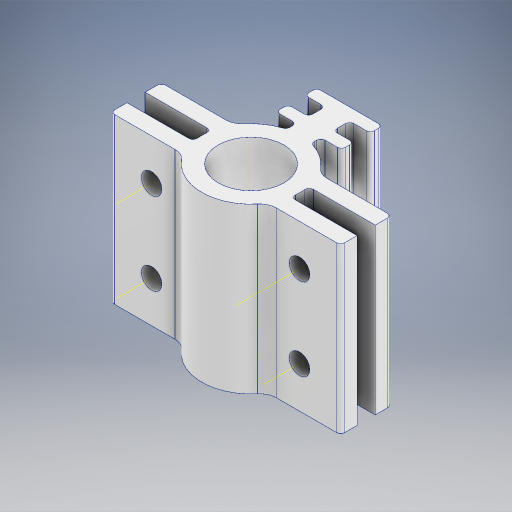
# Autodesk Inventor part: link7
Saved by Autodesk Inventor 2024.1 (Build 281209000, 209)
## iProperties
Created: 2023-09-09
Part Number: link7
Material: Aluminum 6061
Document SubType Name: Modeling
Designer: Camilo
Density: 2.7 g/cm^3
Appearance: Aluminum - Flat
Mass: 0.783285 g
Surface Area: 5.56806 cm^2
Volume: 0.290105 cm^3
Author: Camilo
Autodesk Inventor part; units mm, degrees
ref_plane "YZ Plane" through (0, 0, 0) normal (1, 0, 0) x (0, 1, 0)
ref_plane "XZ Plane" through (0, 0, 0) normal (0, 1, 0) x (-1, 0, 0)
ref_plane "XY Plane" through (0, 0, 0) normal (0, 0, 1) x (1, 0, 0)
sketch "Sketch2" plane through (0, 0, 0) normal (0, 1, 0) x (-1, 0, 0)
  circle A0 centre (0, 0) radius 4
  line L0 (-14, -10) -> (14, -10)
  line L1 (14, -10) -> (14, 10)
  line L2 (14, 10) -> (-14, 10)
  line L3 (-14, 10) -> (-14, -10)
  line L4 (-14, 0) -> (-14, -1.1)
  line L5 (-14, 0) -> (-14, 1.1)
  line L6 (14, 0) -> (14, -1.1)
  circle A1 centre (0, 0) radius 6
  line L7 (-14, -1.1) -> (-5.8983, -1.1)
  line L8 (-14, 1.1) -> (-5.8983, 1.1)
  line L9 (14, 0) -> (14, 1.1)
  line L10 (14, 1.1) -> (5.8983, 1.1)
  line L11 (14, -1.1) -> (5.8983, -1.1)
  line L12 (-14, -1.1) -> (-6.5, -1.1)
  line L13 (-14, -1.1) -> (-14, -3.1)
  line L14 (-14, -3.1) -> (-5.1371, -3.1)
  line L15 (-14, 1.1) -> (-14, 3.1)
  line L16 (-14, 3.1) -> (-5.1371, 3.1)
  line L17 (14, -1.1) -> (14, -3.1)
  line L18 (14, -3.1) -> (5.1371, -3.1)
  line L19 (14, 1.1) -> (14, 3.1)
  line L20 (14, 3.1) -> (5.1371, 3.1)
  point P0 (0, -10)
  dimension "d50" = 12
  dimension "d37" = 8
  dimension "d38" = 28
  dimension "d39" = 20
  dimension "d40" = 14
  dimension "d41" = 10
  dimension "d42" = 1.1
  dimension "d46" = 1.1
  dimension "d48" = 1.1
  dimension "d51" = 1.1
  dimension "d52" = 7.5
  dimension "d53" = 2
  dimension "d54" = 2
  dimension "d55" = 2
  dimension "d56" = 2
  constraints: 42 end point, 10 point on line, 5 perpendicular, 3 horizontal, 3 midpoint, 3 parallel, 2 coincident, 1 centre point, 10 other
  measures "d37" diameter of A0
  measures "d38" distance of L2.end L1.end
  measures "d39" distance of L1.end L0.end
  measures "d40" horizontal distance of point (0, 0) L0.start
  measures "d41" distance of point (0, -10) point (0, 0)
  measures "d42" distance of L4.start L4.end
  measures "d46" distance of L4.start L5.end
  measures "d48" distance of L6.start L6.end
  measures "d51" distance of L6.start L9.end
  measures "d52" distance of L4.end L12.end
  measures "d53" distance of L4.end L13.end
  measures "d54" distance of L5.end L15.end
  measures "d55" distance of L6.end L17.end
  measures "d56" distance of L9.end L19.end
extrude "Extrusion5" add sketch "Sketch2" along normal mid plane 20 contours L3 L7 A1 L14 | L18 A1 L11 L1 | A1 | L3 L16 A1 L8 | L10 A1 L20 L1
sketch "Sketch3" plane through (0, 0, 0) normal (0, 0, 1) x (1, 0, 0)
  line L0 (14, 10) -> (5.1371, 10) projected
  line L1 (14, 10) -> (9, 10)
  line L2 (9, 10) -> (9, 5)
  line L3 (9, 5) -> (14, 5)
  line L4 (14, 5) -> (14, 10)
  circle A0 centre (9, 5) radius 1.25
  line L5 (5.1371, 10) -> (-5.1371, 10) projected
  line L6 (0, 10) -> (0, -10)
  line L7 (4, -10) -> (-4, -10) projected
  line L8 (-14, -10) -> (-14, 10) projected
  line L9 (-14, 0) -> (14, 0)
  line L10 (14, -10) -> (14, 10) projected
  circle A1 centre (9, -5) radius 1.25
  circle A2 centre (-9, 5) radius 1.25
  circle A3 centre (-9, -5) radius 1.25
  point P0 (0, 0)
  dimension "d59" = 5
  dimension "d60" = 5
  dimension "d61" = 2.5
  constraints: 12 end point, 4 centre point, 4 midpoint, 3 symmetric about line, 2 parallel, 1 coincident, 1 horizontal, 1 perpendicular, 3 other
  measures "d59" distance of L3.end L2.end
  measures "d60" distance of L2.end L1.end
  measures "d61" diameter of A0
extrude "Extrusion6" cut sketch "Sketch3" along normal mid plane 20 contours A0 L3 L2 | L2 L3 A0 | A1 | A2 | A3
fillet "Face Fillet1" radius 2 1 edges at (5.1371, 0, -3.1)
fillet "Face Fillet2" radius 2 1 edges at (-5.1371, 0, -3.1)
fillet "Face Fillet3" radius 2 1 edges at (-5.1371, 0, 3.1)
fillet "Face Fillet4" radius 2 1 edges at (5.1371, 0, 3.1)
fillet "Face Fillet5" radius 0.5 1 edges at (-5.8983, 0, -1.1)
fillet "Face Fillet6" radius 0.5 1 edges at (-5.8983, 0, 1.1)
fillet "Face Fillet7" radius 0.5 1 edges at (5.8983, 0, -1.1)
fillet "Face Fillet8" radius 0.5 1 edges at (5.8983, 0, 1.1)
sketch "Sketch4" plane through (0, 10, 0) normal (0, 1, 0) x (1, 0, 0)
  circle A0 centre (0, 0) radius 6
  line L0 (0, 6) -> (0, 7)
  line L1 (0, 7) -> (1.5, 7)
  line L2 (0, 7) -> (-1.5, 7)
  line L3 (1.5, 7) -> (1.5, 5.8095)
  line L4 (-1.5, 7) -> (-1.5, 5.8095)
  line L5 (0, 7) -> (4, 7)
  line L6 (4, 7) -> (-4, 7)
  line L7 (-4, 7) -> (-4, 8.5)
  line L8 (-4, 8.5) -> (4, 8.5)
  line L9 (4, 8.5) -> (4, 7)
  line L10 (0, 8.5) -> (1.5, 8.5)
  line L11 (1.5, 8.5) -> (-1.5, 8.5)
  line L12 (-1.5, 8.5) -> (-1.5, 10.5)
  line L13 (-1.5, 10.5) -> (1.5, 10.5)
  line L14 (1.5, 10.5) -> (1.5, 8.5)
  line L15 (-1.5, 10.5) -> (-4, 10.5)
  line L16 (-4, 10.5) -> (4, 10.5)
  line L17 (4, 10.5) -> (4, 12)
  line L18 (4, 12) -> (-4, 12)
  line L19 (-4, 12) -> (-4, 10.5)
  dimension "d72" = 1
  dimension "d73" = 1.5
  dimension "d74" = 1.5
  dimension "d75" = 4
  dimension "d76" = 8
  dimension "d77" = 1.5
  dimension "d78" = 2
  dimension "d79" = 8
  dimension "d80" = 1.5
  dimension "d82" = 12
  constraints: 40 end point, 7 horizontal, 7 parallel, 3 perpendicular, 3 point on circle, 2 vertical, 1 centre point, 1 coincident, 1 midpoint, 1 point on line
  measures "d72" distance of L0.start L0.end
  measures "d73" distance of L0.end L1.end
  measures "d74" distance of L0.end L2.end
  measures "d75" distance of L0.end L5.end
  measures "d76" distance of L7.end L8.end
  measures "d77" distance of L6.end L7.end
  measures "d78" distance of L11.end L12.end
  measures "d79" distance of L18.end L17.end
  measures "d80" distance of L17.end L16.end
  measures "d82" diameter of A0
extrude "Extrusion7" add sketch "Sketch4" against normal blind 20 contours A0 L0 L1 L3 | L4 L2 L0 A0 | L1 L2 L6 L7 L8 L9 L5 | L8 L12 L13 L14 | L13 L15 L19 L18 L17 L16
fillet "Face Fillet9" radius 0.5 1 edges at (1.5, 0, -5.8095)
fillet "Face Fillet10" radius 0.5 1 edges at (1.5, 0, -7)
fillet "Face Fillet11" radius 0.5 1 edges at (-1.5, 0, -5.8095)
fillet "Face Fillet12" radius 0.5 1 edges at (-1.5, 0, -7)
fillet "Face Fillet13" radius 0.5 1 edges at (-1.5, 0, -8.5)
fillet "Face Fillet14" radius 0.5 1 edges at (-1.5, 0, -10.5)
fillet "Face Fillet15" radius 0.5 1 edges at (1.5, 0, -8.5)
fillet "Face Fillet16" radius 0.5 1 edges at (1.5, 0, -10.5)
fillet "Face Fillet17" radius 0.5 1 edges at (4, 0, -7)
fillet "Face Fillet18" radius 0.5 1 edges at (4, 0, -8.5)
fillet "Face Fillet19" radius 0.5 1 edges at (-4, 0, -8.5)
fillet "Face Fillet20" radius 0.5 1 edges at (-4, 0, -7)
fillet "Face Fillet21" radius 0.5 1 edges at (-4, 0, -10.5)
fillet "Face Fillet22" radius 0.5 1 edges at (-4, 0, -12)
fillet "Face Fillet23" radius 0.5 1 edges at (4, 0, -10.5)
fillet "Face Fillet24" radius 0.5 1 edges at (4, 0, -12)
fillet "Face Fillet25" radius 0.5 1 edges at (14, 0, 3.1)
fillet "Face Fillet26" radius 0.5 1 edges at (14, 0, -3.1)
fillet "Face Fillet27" radius 0.5 1 edges at (-14, 0, 3.1)
fillet "Face Fillet28" radius 0.5 1 edges at (-14, 0, -3.1)
body "Solid2"
